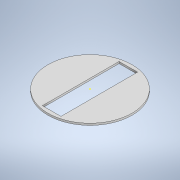
# Autodesk Inventor part: Деталь1
Saved by Autodesk Inventor 2020 (Build 240168000, 168)
## iProperties
Created: 2019-12-15
Part Number: Деталь1
Material: Типовые
Document SubType Name: Modeling
Designer: Валерий
Density: 1 g/cm^3
Appearance: По умолчанию
Author: Валерий
Autodesk Inventor part; units mm, degrees
ref_plane "YZ Plane" through (0, 0, 0) normal (1, 0, 0) x (0, 1, 0)
ref_plane "XZ Plane" through (0, 0, 0) normal (0, 1, 0) x (-1, 0, 0)
ref_plane "XY Plane" through (0, 0, 0) normal (0, 0, 1) x (1, 0, 0)
sketch "Эскиз1" plane through (0, 0, 0) normal (0, 1, 0) x (-1, 0, 0)
  circle A0 centre (0, 0) radius 68
  dimension "d0" = 136
  constraints: 1 centre point, 1 coincident
  measures "d0" diameter of A0
extrude "Выдавливание1" add sketch "Эскиз1" along normal blind 3
sketch "Эскиз2" plane through (0, 3, 0) normal (0, 1, 0) x (1, 0, 0)
  line L0 (15, -62) -> (-15, -62)
  line L1 (-15, -62) -> (-15, 62)
  line L2 (-15, 62) -> (15, 62)
  line L3 (15, 62) -> (15, -62)
  line L4 (15, -62) -> (-15, 62) construction
  line L5 (-15, -62) -> (15, 62) construction
  point P0 (0, 0)
  dimension "d3" = 30
  dimension "d4" = 124
  constraints: 12 end point, 2 midpoint, 2 parallel, 1 horizontal, 1 perpendicular
  measures "d3" distance of L1.end L2.end
  measures "d4" distance of L0.end L1.end
extrude "Выдавливание2" cut sketch "Эскиз2" against normal blind 3
sketch "Эскиз3" plane through (0, 3, 0) normal (0, 1, 0) x (1, 0, 0)
  point P0 (0, 0)
